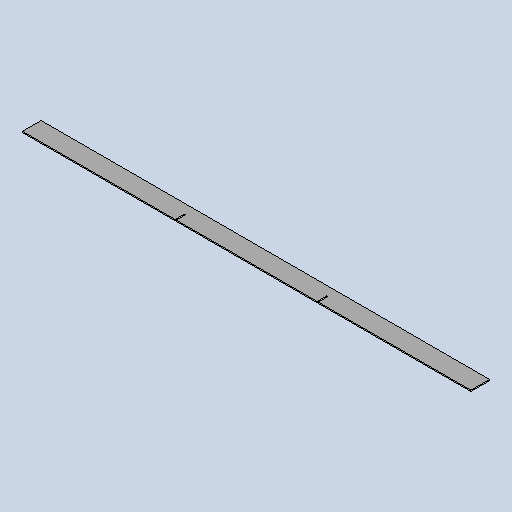
# Autodesk Inventor part: MSC 106 rib cone
Saved by Autodesk Inventor 2025 (Build 290162010, 162A)
## iProperties
Created: 2024-06-26
Part Number: MSC 106 rib cone
Material: Stainless Steel
Document SubType Name: Sheet Metal
Designer: pokla
Density: 8 g/cm^3
Sheet Metal Rule: AISI304 3mm Die 32
Appearance: Default
Stock Number: МОО 106 шпангоут конус
Author: pokla
Autodesk Inventor part; units mm, degrees
ref_plane "YZ Plane" through (0, 0, 0) normal (1, 0, 0) x (0, 1, 0)
ref_plane "XZ Plane" through (0, 0, 0) normal (0, 1, 0) x (-1, 0, 0)
ref_plane "XY Plane" through (0, 0, 0) normal (0, 0, 1) x (1, 0, 0)
sketch "Sketch1" plane through (0, 0, 0) normal (0, 0, 1) x (1, 0, 0)
  line L0 (-600, 0) -> (600, 0)
  line L1 (-600, 0) -> (-600, 50)
  line L2 (-600, 50) -> (600, 50)
  line L3 (600, 50) -> (600, 0)
  circle A0 centre (-600, 0) radius 25
  circle A1 centre (600, 0) radius 25
  line L4 (600, 0) -> (644.2345, 16.1001)
  line L5 (644.2345, 16.1001) -> (635, 50)
  line L6 (635, 50) -> (600, 50)
  point P0 (0, 0)
  point P1 (0, 0)
  point P2 (-600, 25)
  point P3 (-575, 0)
  point P4 (575, 0)
  point P5 (600, 25)
  point P6 (623.4923, 8.5505)
  dimension "d18" = 50
  dimension "d19" = 1200
  dimension "d25" = 50
  dimension "d26" = 50
  dimension "d39" = 70
  dimension "d40" = 35
  measures "d18" distance of L2.end L0.end
  measures "d19" distance of L0.start L0.end
  measures "d25" diameter of A0
  measures "d26" diameter of A1
  measures "d39" angle of L3 L4
  measures "d40" distance of L2.end L5.end
extrude "Plate2" add sketch "Sketch1" against normal blind 3 contours L1 A0 L0 | A0 L1 L2 L3 A1 L0 | A1 L3 L0 picked at (-598.1457, 16.4577)
sketch "Sketch3" plane through (0, 0, 0) normal (0, 0, 1) x (1, 0, 0)
  line L0 (-190, 0) -> (-190, 50) construction
  line L1 (600, 50) -> (-600, 50) projected
  line L2 (-600, 50) -> (-600, 0) projected
  line L3 (-191.5, 26) -> (-188.5, 26)
  line L4 (-188.5, 26) -> (-188.5, 0)
  line L5 (-188.5, 0) -> (-191.5, 0)
  line L6 (-191.5, 0) -> (-191.5, 26)
  line L7 (-600, 0) -> (600, 0) projected
  line L8 (190, 50) -> (190, 0) construction
  line L9 (188.5, 26) -> (191.5, 26)
  line L10 (191.5, 26) -> (191.5, 0)
  line L11 (191.5, 0) -> (188.5, 0)
  line L12 (188.5, 0) -> (188.5, 26)
  point P0 (0, 0)
  point P1 (-550, 25)
  point P2 (-525, 0)
  point P3 (525, 0)
  point P4 (0, 0)
  point P5 (0, 0)
  point P6 (191.5, 0)
  point P7 (585, 50)
  dimension "d28" = 3
  dimension "d29" = 26
  dimension "d35" = 190
  dimension "d36" = 190
  dimension "d37" = 3
  dimension "d38" = 26
  constraints: 20 end point, 4 parallel, 2 horizontal, 2 midpoint, 2 perpendicular, 2 point on line, 2 vertical, 6 other
  measures "d28" distance of L4.end L5.end
  measures "d29" distance of L3.end L4.end
  measures "d35" distance from line of point (0, 0) L0
  measures "d36" distance from line of point (0, 0) L8
  measures "d37" distance of L10.end L11.end
  measures "d38" distance of L9.end L10.end
extrude "Extrusion2" cut sketch "Sketch3" against normal through all
equation "\"d28\" = Thickness"
equation "\"d36\" = d35"
equation "\"d37\" = Thickness"
equation "\"d38\" = d29"
equation "\"d20\" = Thickness"
equation "\"BendReliefWidth\" = Thickness"
equation "\"BendReliefDepth\" = 0.5 * Thickness"
equation "\"CornerReliefSize\" = 4 * Thickness"
equation "\"MinimumRemnant\" = 2 * Thickness"
equation "\"TransitionRadius\" = BendRadius"
equation "\"JacobiRadiusSize\" = BendRadius"
equation "\"GapSize\" = Thickness"
equation "\"Thickness\" = 3"
equation "\"BendRadius\" = 5"
body "Solid2"
